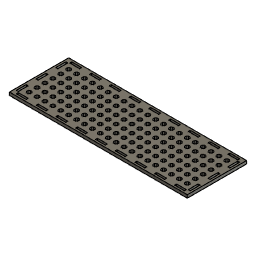
Modular Test Bench - Jumper Board v1 (Autodesk Fusion 360 design; units mm, degrees)
Autodesk Fusion 360 part; units mm, degrees
(part 1 of 2)
sketch "Sketch1" plane through (0, 0, 0) normal (0, 1, 0) x (1, 0, 0)
  line L0 (0, 0) -> (180, 0)
  line L1 (180, 0) -> (180, 60)
  line L2 (180, 60) -> (0, 60)
  line L3 (0, 60) -> (0, 0)
  dimension "d1" = 60
  dimension "d2" = 180
  constraint horizontal L0
  constraint vertical L1
  constraint horizontal L2
  constraint vertical L3
  constraint coincident L0.start L3.end
  measures "d1" distance of L0.start L2.end
  measures "d2" distance of L0.start L0.end
extrude "Extrude1" add sketch "Sketch1" along normal blind 3
sketch "Sketch2" plane through (0, 3, 0) normal (0, 1, 0) x (-1, 0, 0)
  line L0 (0, -60) -> (0, 0)
  line L1 (0, 0) -> (-180, 0)
  line L2 (-180, 0) -> (-180, -60)
  line L3 (-180, -60) -> (0, -60)
  line L4 (-5, -2) -> (-15, -2)
  line L5 (-15, -2) -> (-15, -4)
  line L6 (-15, -4) -> (-5, -4)
  line L7 (-5, -4) -> (-5, -2)
  line L8 (-25, -2) -> (-35, -2)
  line L9 (-25, -4) -> (-25, -2)
  line L10 (-35, -2) -> (-35, -4)
  line L11 (-35, -4) -> (-25, -4)
  line L12 (-45, -2) -> (-55, -2)
  line L13 (-45, -4) -> (-45, -2)
  line L14 (-55, -2) -> (-55, -4)
  line L15 (-55, -4) -> (-45, -4)
  line L16 (-65, -2) -> (-75, -2)
  line L17 (-65, -4) -> (-65, -2)
  line L18 (-75, -2) -> (-75, -4)
  line L19 (-75, -4) -> (-65, -4)
  line L20 (-85, -2) -> (-95, -2)
  line L21 (-85, -4) -> (-85, -2)
  line L22 (-95, -2) -> (-95, -4)
  line L23 (-95, -4) -> (-85, -4)
  line L24 (-105, -2) -> (-115, -2)
  line L25 (-105, -4) -> (-105, -2)
  line L26 (-115, -2) -> (-115, -4)
  line L27 (-115, -4) -> (-105, -4)
  line L28 (-125, -2) -> (-135, -2)
  line L29 (-125, -4) -> (-125, -2)
  line L30 (-135, -2) -> (-135, -4)
  line L31 (-135, -4) -> (-125, -4)
  line L32 (-145, -2) -> (-155, -2)
  line L33 (-145, -4) -> (-145, -2)
  line L34 (-155, -2) -> (-155, -4)
  line L35 (-155, -4) -> (-145, -4)
  line L36 (-165, -2) -> (-175, -2)
  line L37 (-165, -4) -> (-165, -2)
  line L38 (-175, -2) -> (-175, -4)
  line L39 (-175, -4) -> (-165, -4)
  line L40 (-5, -56) -> (-15, -56)
  line L41 (-5, -58) -> (-5, -56)
  line L42 (-15, -56) -> (-15, -58)
  line L43 (-15, -58) -> (-5, -58)
  line L44 (-25, -56) -> (-35, -56)
  line L45 (-25, -58) -> (-25, -56)
  line L46 (-35, -56) -> (-35, -58)
  line L47 (-35, -58) -> (-25, -58)
  line L48 (-45, -56) -> (-55, -56)
  line L49 (-45, -58) -> (-45, -56)
  line L50 (-55, -56) -> (-55, -58)
  line L51 (-55, -58) -> (-45, -58)
  line L52 (-65, -56) -> (-75, -56)
  line L53 (-65, -58) -> (-65, -56)
  line L54 (-75, -56) -> (-75, -58)
  line L55 (-75, -58) -> (-65, -58)
  line L56 (-85, -56) -> (-95, -56)
  line L57 (-85, -58) -> (-85, -56)
  line L58 (-95, -56) -> (-95, -58)
  line L59 (-95, -58) -> (-85, -58)
  line L60 (-105, -56) -> (-115, -56)
  line L61 (-105, -58) -> (-105, -56)
  line L62 (-115, -56) -> (-115, -58)
  line L63 (-115, -58) -> (-105, -58)
  line L64 (-125, -56) -> (-135, -56)
  line L65 (-125, -58) -> (-125, -56)
  line L66 (-135, -56) -> (-135, -58)
  line L67 (-135, -58) -> (-125, -58)
  line L68 (-145, -56) -> (-155, -56)
  line L69 (-145, -58) -> (-145, -56)
  line L70 (-155, -56) -> (-155, -58)
  line L71 (-155, -58) -> (-145, -58)
  line L72 (-165, -56) -> (-175, -56)
  line L73 (-165, -58) -> (-165, -56)
  line L74 (-175, -56) -> (-175, -58)
  line L75 (-175, -58) -> (-165, -58)
  line L76 (-2, -5) -> (-4, -5)
  line L77 (-4, -5) -> (-4, -15)
  line L78 (-4, -15) -> (-2, -15)
  line L79 (-2, -15) -> (-2, -5)
  line L80 (-178, -5) -> (-178, -15)
  line L81 (-176, -5) -> (-178, -5)
  line L82 (-176, -15) -> (-176, -5)
  line L83 (-178, -15) -> (-176, -15)
  line L84 (-4, -25) -> (-4, -35)
  line L85 (-2, -25) -> (-4, -25)
  line L86 (-2, -35) -> (-2, -25)
  line L87 (-4, -35) -> (-2, -35)
  line L88 (-178, -25) -> (-178, -35)
  line L89 (-176, -25) -> (-178, -25)
  line L90 (-176, -35) -> (-176, -25)
  line L91 (-178, -35) -> (-176, -35)
  line L92 (-4, -45) -> (-4, -55)
  line L93 (-2, -45) -> (-4, -45)
  line L94 (-2, -55) -> (-2, -45)
  line L95 (-4, -55) -> (-2, -55)
  line L96 (-178, -45) -> (-178, -55)
  line L97 (-176, -45) -> (-178, -45)
  line L98 (-176, -55) -> (-176, -45)
  line L99 (-178, -55) -> (-176, -55)
  line L100 (-12.0079, -50.8092) -> (-10.8476, -51.992)
  line L101 (-10.8476, -51.992) -> (-9.1908, -52.0079)
  line L102 (-9.1908, -52.0079) -> (-8.008, -50.8476)
  line L103 (-8.008, -50.8476) -> (-7.9921, -49.1908)
  line L104 (-7.9921, -49.1908) -> (-9.1524, -48.008)
  line L105 (-9.1524, -48.008) -> (-10.8092, -47.9921)
  line L106 (-10.8092, -47.9921) -> (-11.992, -49.1524)
  line L107 (-11.992, -49.1524) -> (-12.0079, -50.8092)
  line L108 (-18.8476, -51.992) -> (-17.1908, -52.0079)
  line L109 (-16.008, -50.8476) -> (-15.9921, -49.1908)
  line L110 (-15.9921, -49.1908) -> (-17.1524, -48.008)
  line L111 (-20.0079, -50.8092) -> (-18.8476, -51.992)
  line L112 (-17.1524, -48.008) -> (-18.8092, -47.9921)
  line L113 (-18.8092, -47.9921) -> (-19.992, -49.1524)
  line L114 (-19.992, -49.1524) -> (-20.0079, -50.8092)
  line L115 (-17.1908, -52.0079) -> (-16.008, -50.8476)
  line L116 (-26.8476, -51.992) -> (-25.1908, -52.0079)
  line L117 (-24.008, -50.8476) -> (-23.9921, -49.1908)
  line L118 (-23.9921, -49.1908) -> (-25.1524, -48.008)
  line L119 (-28.0079, -50.8092) -> (-26.8476, -51.992)
  line L120 (-25.1524, -48.008) -> (-26.8092, -47.9921)
  line L121 (-26.8092, -47.9921) -> (-27.992, -49.1524)
  line L122 (-27.992, -49.1524) -> (-28.0079, -50.8092)
  line L123 (-25.1908, -52.0079) -> (-24.008, -50.8476)
  line L124 (-34.8476, -51.992) -> (-33.1908, -52.0079)
  line L125 (-32.008, -50.8476) -> (-31.9921, -49.1908)
  line L126 (-31.9921, -49.1908) -> (-33.1524, -48.008)
  line L127 (-36.0079, -50.8092) -> (-34.8476, -51.992)
  line L128 (-33.1524, -48.008) -> (-34.8092, -47.9921)
  line L129 (-34.8092, -47.9921) -> (-35.992, -49.1524)
  line L130 (-35.992, -49.1524) -> (-36.0079, -50.8092)
  line L131 (-33.1908, -52.0079) -> (-32.008, -50.8476)
  line L132 (-42.8476, -51.992) -> (-41.1908, -52.0079)
  line L133 (-40.008, -50.8476) -> (-39.9921, -49.1908)
  line L134 (-39.9921, -49.1908) -> (-41.1524, -48.008)
  line L135 (-44.0079, -50.8092) -> (-42.8476, -51.992)
  line L136 (-41.1524, -48.008) -> (-42.8092, -47.9921)
  line L137 (-42.8092, -47.9921) -> (-43.992, -49.1524)
  line L138 (-43.992, -49.1524) -> (-44.0079, -50.8092)
  line L139 (-41.1908, -52.0079) -> (-40.008, -50.8476)
  line L140 (-50.8476, -51.992) -> (-49.1908, -52.0079)
  line L141 (-48.008, -50.8476) -> (-47.9921, -49.1908)
  line L142 (-47.9921, -49.1908) -> (-49.1524, -48.008)
  line L143 (-52.0079, -50.8092) -> (-50.8476, -51.992)
  line L144 (-49.1524, -48.008) -> (-50.8092, -47.9921)
  line L145 (-50.8092, -47.9921) -> (-51.992, -49.1524)
  line L146 (-51.992, -49.1524) -> (-52.0079, -50.8092)
  line L147 (-49.1908, -52.0079) -> (-48.008, -50.8476)
  line L148 (-58.8476, -51.992) -> (-57.1908, -52.0079)
  line L149 (-56.008, -50.8476) -> (-55.9921, -49.1908)
  line L150 (-55.9921, -49.1908) -> (-57.1524, -48.008)
  line L151 (-60.0079, -50.8092) -> (-58.8476, -51.992)
  line L152 (-57.1524, -48.008) -> (-58.8092, -47.9921)
  line L153 (-58.8092, -47.9921) -> (-59.992, -49.1524)
  line L154 (-59.992, -49.1524) -> (-60.0079, -50.8092)
  line L155 (-57.1908, -52.0079) -> (-56.008, -50.8476)
  line L156 (-66.8476, -51.992) -> (-65.1908, -52.0079)
  line L157 (-64.008, -50.8476) -> (-63.9921, -49.1908)
  line L158 (-63.9921, -49.1908) -> (-65.1524, -48.008)
  line L159 (-68.0079, -50.8092) -> (-66.8476, -51.992)
  line L160 (-65.1524, -48.008) -> (-66.8092, -47.9921)
  line L161 (-66.8092, -47.9921) -> (-67.992, -49.1524)
  line L162 (-67.992, -49.1524) -> (-68.0079, -50.8092)
  line L163 (-65.1908, -52.0079) -> (-64.008, -50.8476)
  line L164 (-74.8476, -51.992) -> (-73.1908, -52.0079)
  line L165 (-72.008, -50.8476) -> (-71.9921, -49.1908)
  line L166 (-71.9921, -49.1908) -> (-73.1524, -48.008)
  line L167 (-76.0079, -50.8092) -> (-74.8476, -51.992)
  line L168 (-73.1524, -48.008) -> (-74.8092, -47.9921)
  line L169 (-74.8092, -47.9921) -> (-75.992, -49.1524)
  line L170 (-75.992, -49.1524) -> (-76.0079, -50.8092)
  line L171 (-73.1908, -52.0079) -> (-72.008, -50.8476)
  line L172 (-82.8476, -51.992) -> (-81.1908, -52.0079)
  line L173 (-80.008, -50.8476) -> (-79.9921, -49.1908)
  line L174 (-79.9921, -49.1908) -> (-81.1524, -48.008)
  line L175 (-84.0079, -50.8092) -> (-82.8476, -51.992)
  line L176 (-81.1524, -48.008) -> (-82.8092, -47.9921)
  line L177 (-82.8092, -47.9921) -> (-83.992, -49.1524)
  line L178 (-83.992, -49.1524) -> (-84.0079, -50.8092)
  line L179 (-81.1908, -52.0079) -> (-80.008, -50.8476)
  line L180 (-90.8476, -51.992) -> (-89.1908, -52.0079)
  line L181 (-88.008, -50.8476) -> (-87.9921, -49.1908)
  line L182 (-87.9921, -49.1908) -> (-89.1524, -48.008)
  line L183 (-92.0079, -50.8092) -> (-90.8476, -51.992)
  line L184 (-89.1524, -48.008) -> (-90.8092, -47.9921)
  line L185 (-90.8092, -47.9921) -> (-91.992, -49.1524)
  line L186 (-91.992, -49.1524) -> (-92.0079, -50.8092)
  line L187 (-89.1908, -52.0079) -> (-88.008, -50.8476)
  line L188 (-98.8476, -51.992) -> (-97.1908, -52.0079)
  line L189 (-96.008, -50.8476) -> (-95.9921, -49.1908)
  line L190 (-95.9921, -49.1908) -> (-97.1524, -48.008)
  line L191 (-100.0079, -50.8092) -> (-98.8476, -51.992)
  line L192 (-97.1524, -48.008) -> (-98.8092, -47.9921)
  line L193 (-98.8092, -47.9921) -> (-99.992, -49.1524)
  line L194 (-99.992, -49.1524) -> (-100.0079, -50.8092)
  line L195 (-97.1908, -52.0079) -> (-96.008, -50.8476)
  line L196 (-106.8476, -51.992) -> (-105.1908, -52.0079)
  line L197 (-104.008, -50.8476) -> (-103.9921, -49.1908)
  line L198 (-103.9921, -49.1908) -> (-105.1524, -48.008)
  line L199 (-108.0079, -50.8092) -> (-106.8476, -51.992)
  line L200 (-105.1524, -48.008) -> (-106.8092, -47.9921)
  line L201 (-106.8092, -47.9921) -> (-107.992, -49.1524)
  line L202 (-107.992, -49.1524) -> (-108.0079, -50.8092)
  line L203 (-105.1908, -52.0079) -> (-104.008, -50.8476)
  line L204 (-114.8476, -51.992) -> (-113.1908, -52.0079)
  line L205 (-112.008, -50.8476) -> (-111.9921, -49.1908)
  line L206 (-111.9921, -49.1908) -> (-113.1524, -48.008)
  line L207 (-116.0079, -50.8092) -> (-114.8476, -51.992)
  line L208 (-113.1524, -48.008) -> (-114.8092, -47.9921)
  line L209 (-114.8092, -47.9921) -> (-115.992, -49.1524)
  line L210 (-115.992, -49.1524) -> (-116.0079, -50.8092)
  line L211 (-113.1908, -52.0079) -> (-112.008, -50.8476)
  line L212 (-122.8476, -51.992) -> (-121.1908, -52.0079)
  line L213 (-120.008, -50.8476) -> (-119.9921, -49.1908)
  line L214 (-119.9921, -49.1908) -> (-121.1524, -48.008)
  line L215 (-124.0079, -50.8092) -> (-122.8476, -51.992)
  line L216 (-121.1524, -48.008) -> (-122.8092, -47.9921)
  line L217 (-122.8092, -47.9921) -> (-123.992, -49.1524)
  line L218 (-123.992, -49.1524) -> (-124.0079, -50.8092)
  line L219 (-121.1908, -52.0079) -> (-120.008, -50.8476)
  line L220 (-130.8476, -51.992) -> (-129.1908, -52.0079)
  line L221 (-128.008, -50.8476) -> (-127.9921, -49.1908)
  line L222 (-127.9921, -49.1908) -> (-129.1524, -48.008)
  line L223 (-132.0079, -50.8092) -> (-130.8476, -51.992)
  line L224 (-129.1524, -48.008) -> (-130.8092, -47.9921)
  line L225 (-130.8092, -47.9921) -> (-131.992, -49.1524)
  line L226 (-131.992, -49.1524) -> (-132.0079, -50.8092)
  line L227 (-129.1908, -52.0079) -> (-128.008, -50.8476)
  line L228 (-138.8476, -51.992) -> (-137.1908, -52.0079)
  line L229 (-136.008, -50.8476) -> (-135.9921, -49.1908)
  line L230 (-135.9921, -49.1908) -> (-137.1524, -48.008)
  line L231 (-140.0079, -50.8092) -> (-138.8476, -51.992)
  line L232 (-137.1524, -48.008) -> (-138.8092, -47.9921)
  line L233 (-138.8092, -47.9921) -> (-139.992, -49.1524)
  line L234 (-139.992, -49.1524) -> (-140.0079, -50.8092)
  line L235 (-137.1908, -52.0079) -> (-136.008, -50.8476)
  line L236 (-146.8476, -51.992) -> (-145.1908, -52.0079)
  line L237 (-144.008, -50.8476) -> (-143.9921, -49.1908)
  line L238 (-143.9921, -49.1908) -> (-145.1524, -48.008)
  line L239 (-148.0079, -50.8092) -> (-146.8476, -51.992)
  line L240 (-145.1524, -48.008) -> (-146.8092, -47.9921)
  line L241 (-146.8092, -47.9921) -> (-147.992, -49.1524)
  line L242 (-147.992, -49.1524) -> (-148.0079, -50.8092)
  line L243 (-145.1908, -52.0079) -> (-144.008, -50.8476)
  line L244 (-154.8476, -51.992) -> (-153.1908, -52.0079)
  line L245 (-152.008, -50.8476) -> (-151.9921, -49.1908)
  line L246 (-151.9921, -49.1908) -> (-153.1524, -48.008)
  line L247 (-156.0079, -50.8092) -> (-154.8476, -51.992)
  line L248 (-153.1524, -48.008) -> (-154.8092, -47.9921)
  line L249 (-154.8092, -47.9921) -> (-155.992, -49.1524)
  line L250 (-155.992, -49.1524) -> (-156.0079, -50.8092)
  line L251 (-153.1908, -52.0079) -> (-152.008, -50.8476)
  line L252 (-162.8476, -51.992) -> (-161.1908, -52.0079)
  line L253 (-160.008, -50.8476) -> (-159.9921, -49.1908)
  line L254 (-159.9921, -49.1908) -> (-161.1524, -48.008)
  line L255 (-164.0079, -50.8092) -> (-162.8476, -51.992)
  line L256 (-161.1524, -48.008) -> (-162.8092, -47.9921)
  line L257 (-162.8092, -47.9921) -> (-163.992, -49.1524)
  line L258 (-163.992, -49.1524) -> (-164.0079, -50.8092)
  line L259 (-161.1908, -52.0079) -> (-160.008, -50.8476)
  line L260 (-170.8476, -51.992) -> (-169.1908, -52.0079)
  line L261 (-168.008, -50.8476) -> (-167.9921, -49.1908)
  line L262 (-167.9921, -49.1908) -> (-169.1524, -48.008)
  line L263 (-172.0079, -50.8092) -> (-170.8476, -51.992)
  line L264 (-169.1524, -48.008) -> (-170.8092, -47.9921)
  line L265 (-170.8092, -47.9921) -> (-171.992, -49.1524)
  line L266 (-171.992, -49.1524) -> (-172.0079, -50.8092)
  line L267 (-169.1908, -52.0079) -> (-168.008, -50.8476)
  line L268 (-10.8476, -43.992) -> (-9.1908, -44.0079)
  line L269 (-8.008, -42.8476) -> (-7.9921, -41.1908)
  line L270 (-7.9921, -41.1908) -> (-9.1524, -40.008)
  line L271 (-12.0079, -42.8092) -> (-10.8476, -43.992)
  line L272 (-9.1524, -40.008) -> (-10.8092, -39.9921)
  line L273 (-10.8092, -39.9921) -> (-11.992, -41.1524)
  line L274 (-11.992, -41.1524) -> (-12.0079, -42.8092)
  line L275 (-9.1908, -44.0079) -> (-8.008, -42.8476)
  line L276 (-18.8476, -43.992) -> (-17.1908, -44.0079)
  line L277 (-16.008, -42.8476) -> (-15.9921, -41.1908)
  line L278 (-15.9921, -41.1908) -> (-17.1524, -40.008)
  line L279 (-20.0079, -42.8092) -> (-18.8476, -43.992)
  line L280 (-17.1524, -40.008) -> (-18.8092, -39.9921)
  line L281 (-18.8092, -39.9921) -> (-19.992, -41.1524)
  line L282 (-19.992, -41.1524) -> (-20.0079, -42.8092)
  line L283 (-17.1908, -44.0079) -> (-16.008, -42.8476)
  line L284 (-26.8476, -43.992) -> (-25.1908, -44.0079)
  line L285 (-24.008, -42.8476) -> (-23.9921, -41.1908)
  line L286 (-23.9921, -41.1908) -> (-25.1524, -40.008)
  line L287 (-28.0079, -42.8092) -> (-26.8476, -43.992)
  line L288 (-25.1524, -40.008) -> (-26.8092, -39.9921)
  line L289 (-26.8092, -39.9921) -> (-27.992, -41.1524)
  line L290 (-27.992, -41.1524) -> (-28.0079, -42.8092)
  line L291 (-25.1908, -44.0079) -> (-24.008, -42.8476)
  line L292 (-34.8476, -43.992) -> (-33.1908, -44.0079)
  line L293 (-32.008, -42.8476) -> (-31.9921, -41.1908)
  line L294 (-31.9921, -41.1908) -> (-33.1524, -40.008)
  line L295 (-36.0079, -42.8092) -> (-34.8476, -43.992)
  line L296 (-33.1524, -40.008) -> (-34.8092, -39.9921)
  line L297 (-34.8092, -39.9921) -> (-35.992, -41.1524)
  line L298 (-35.992, -41.1524) -> (-36.0079, -42.8092)
  line L299 (-33.1908, -44.0079) -> (-32.008, -42.8476)
  line L300 (-42.8476, -43.992) -> (-41.1908, -44.0079)
  line L301 (-40.008, -42.8476) -> (-39.9921, -41.1908)
  line L302 (-39.9921, -41.1908) -> (-41.1524, -40.008)
  line L303 (-44.0079, -42.8092) -> (-42.8476, -43.992)
  line L304 (-41.1524, -40.008) -> (-42.8092, -39.9921)
  line L305 (-42.8092, -39.9921) -> (-43.992, -41.1524)
  line L306 (-43.992, -41.1524) -> (-44.0079, -42.8092)
  line L307 (-41.1908, -44.0079) -> (-40.008, -42.8476)
  line L308 (-50.8476, -43.992) -> (-49.1908, -44.0079)
  line L309 (-48.008, -42.8476) -> (-47.9921, -41.1908)
  line L310 (-47.9921, -41.1908) -> (-49.1524, -40.008)
  line L311 (-52.0079, -42.8092) -> (-50.8476, -43.992)
  line L312 (-49.1524, -40.008) -> (-50.8092, -39.9921)
  line L313 (-50.8092, -39.9921) -> (-51.992, -41.1524)
  line L314 (-51.992, -41.1524) -> (-52.0079, -42.8092)
  line L315 (-49.1908, -44.0079) -> (-48.008, -42.8476)
  line L316 (-58.8476, -43.992) -> (-57.1908, -44.0079)
  line L317 (-56.008, -42.8476) -> (-55.9921, -41.1908)
  line L318 (-55.9921, -41.1908) -> (-57.1524, -40.008)
  line L319 (-60.0079, -42.8092) -> (-58.8476, -43.992)
  line L320 (-57.1524, -40.008) -> (-58.8092, -39.9921)
  line L321 (-58.8092, -39.9921) -> (-59.992, -41.1524)
  line L322 (-59.992, -41.1524) -> (-60.0079, -42.8092)
  line L323 (-57.1908, -44.0079) -> (-56.008, -42.8476)
  line L324 (-66.8476, -43.992) -> (-65.1908, -44.0079)
  line L325 (-64.008, -42.8476) -> (-63.9921, -41.1908)
  line L326 (-63.9921, -41.1908) -> (-65.1524, -40.008)
  line L327 (-68.0079, -42.8092) -> (-66.8476, -43.992)
  line L328 (-65.1524, -40.008) -> (-66.8092, -39.9921)
  line L329 (-66.8092, -39.9921) -> (-67.992, -41.1524)
  line L330 (-67.992, -41.1524) -> (-68.0079, -42.8092)
  line L331 (-65.1908, -44.0079) -> (-64.008, -42.8476)
  line L332 (-74.8476, -43.992) -> (-73.1908, -44.0079)
  line L333 (-72.008, -42.8476) -> (-71.9921, -41.1908)
  line L334 (-71.9921, -41.1908) -> (-73.1524, -40.008)
  line L335 (-76.0079, -42.8092) -> (-74.8476, -43.992)
  line L336 (-73.1524, -40.008) -> (-74.8092, -39.9921)
  line L337 (-74.8092, -39.9921) -> (-75.992, -41.1524)
  line L338 (-75.992, -41.1524) -> (-76.0079, -42.8092)
  line L339 (-73.1908, -44.0079) -> (-72.008, -42.8476)
  line L340 (-82.8476, -43.992) -> (-81.1908, -44.0079)
  line L341 (-80.008, -42.8476) -> (-79.9921, -41.1908)
  line L342 (-79.9921, -41.1908) -> (-81.1524, -40.008)
  line L343 (-84.0079, -42.8092) -> (-82.8476, -43.992)
  line L344 (-81.1524, -40.008) -> (-82.8092, -39.9921)
  line L345 (-82.8092, -39.9921) -> (-83.992, -41.1524)
  line L346 (-83.992, -41.1524) -> (-84.0079, -42.8092)
  line L347 (-81.1908, -44.0079) -> (-80.008, -42.8476)
  line L348 (-90.8476, -43.992) -> (-89.1908, -44.0079)
  line L349 (-88.008, -42.8476) -> (-87.9921, -41.1908)
  line L350 (-87.9921, -41.1908) -> (-89.1524, -40.008)
  line L351 (-92.0079, -42.8092) -> (-90.8476, -43.992)
  line L352 (-89.1524, -40.008) -> (-90.8092, -39.9921)
  line L353 (-90.8092, -39.9921) -> (-91.992, -41.1524)
  line L354 (-91.992, -41.1524) -> (-92.0079, -42.8092)
  line L355 (-89.1908, -44.0079) -> (-88.008, -42.8476)
  line L356 (-98.8476, -43.992) -> (-97.1908, -44.0079)
  line L357 (-96.008, -42.8476) -> (-95.9921, -41.1908)
  line L358 (-95.9921, -41.1908) -> (-97.1524, -40.008)
  line L359 (-100.0079, -42.8092) -> (-98.8476, -43.992)
  line L360 (-97.1524, -40.008) -> (-98.8092, -39.9921)
  line L361 (-98.8092, -39.9921) -> (-99.992, -41.1524)
  line L362 (-99.992, -41.1524) -> (-100.0079, -42.8092)
  line L363 (-97.1908, -44.0079) -> (-96.008, -42.8476)
  line L364 (-106.8476, -43.992) -> (-105.1908, -44.0079)
  line L365 (-104.008, -42.8476) -> (-103.9921, -41.1908)
  line L366 (-103.9921, -41.1908) -> (-105.1524, -40.008)
  line L367 (-108.0079, -42.8092) -> (-106.8476, -43.992)
  line L368 (-105.1524, -40.008) -> (-106.8092, -39.9921)
  line L369 (-106.8092, -39.9921) -> (-107.992, -41.1524)
  line L370 (-107.992, -41.1524) -> (-108.0079, -42.8092)
  line L371 (-105.1908, -44.0079) -> (-104.008, -42.8476)
  line L372 (-114.8476, -43.992) -> (-113.1908, -44.0079)
  line L373 (-112.008, -42.8476) -> (-111.9921, -41.1908)
  line L374 (-111.9921, -41.1908) -> (-113.1524, -40.008)
  line L375 (-116.0079, -42.8092) -> (-114.8476, -43.992)
  line L376 (-113.1524, -40.008) -> (-114.8092, -39.9921)
  line L377 (-114.8092, -39.9921) -> (-115.992, -41.1524)
  line L378 (-115.992, -41.1524) -> (-116.0079, -42.8092)
  line L379 (-113.1908, -44.0079) -> (-112.008, -42.8476)
  line L380 (-122.8476, -43.992) -> (-121.1908, -44.0079)
  line L381 (-120.008, -42.8476) -> (-119.9921, -41.1908)
  line L382 (-119.9921, -41.1908) -> (-121.1524, -40.008)
  line L383 (-124.0079, -42.8092) -> (-122.8476, -43.992)
  line L384 (-121.1524, -40.008) -> (-122.8092, -39.9921)
  line L385 (-122.8092, -39.9921) -> (-123.992, -41.1524)
  line L386 (-123.992, -41.1524) -> (-124.0079, -42.8092)
  line L387 (-121.1908, -44.0079) -> (-120.008, -42.8476)
  line L388 (-130.8476, -43.992) -> (-129.1908, -44.0079)
  line L389 (-128.008, -42.8476) -> (-127.9921, -41.1908)
  line L390 (-127.9921, -41.1908) -> (-129.1524, -40.008)
  line L391 (-132.0079, -42.8092) -> (-130.8476, -43.992)
  line L392 (-129.1524, -40.008) -> (-130.8092, -39.9921)
  line L393 (-130.8092, -39.9921) -> (-131.992, -41.1524)
  line L394 (-131.992, -41.1524) -> (-132.0079, -42.8092)
  line L395 (-129.1908, -44.0079) -> (-128.008, -42.8476)
  line L396 (-138.8476, -43.992) -> (-137.1908, -44.0079)
  line L397 (-136.008, -42.8476) -> (-135.9921, -41.1908)
  line L398 (-135.9921, -41.1908) -> (-137.1524, -40.008)
  line L399 (-140.0079, -42.8092) -> (-138.8476, -43.992)
  line L400 (-137.1524, -40.008) -> (-138.8092, -39.9921)
  line L401 (-138.8092, -39.9921) -> (-139.992, -41.1524)
  line L402 (-139.992, -41.1524) -> (-140.0079, -42.8092)
  line L403 (-137.1908, -44.0079) -> (-136.008, -42.8476)
  line L404 (-146.8476, -43.992) -> (-145.1908, -44.0079)
  line L405 (-144.008, -42.8476) -> (-143.9921, -41.1908)
  line L406 (-143.9921, -41.1908) -> (-145.1524, -40.008)
  line L407 (-148.0079, -42.8092) -> (-146.8476, -43.992)
  line L408 (-145.1524, -40.008) -> (-146.8092, -39.9921)
  line L409 (-146.8092, -39.9921) -> (-147.992, -41.1524)
  line L410 (-147.992, -41.1524) -> (-148.0079, -42.8092)
  line L411 (-145.1908, -44.0079) -> (-144.008, -42.8476)
  line L412 (-154.8476, -43.992) -> (-153.1908, -44.0079)
  line L413 (-152.008, -42.8476) -> (-151.9921, -41.1908)
  line L414 (-151.9921, -41.1908) -> (-153.1524, -40.008)
  line L415 (-156.0079, -42.8092) -> (-154.8476, -43.992)
  line L416 (-153.1524, -40.008) -> (-154.8092, -39.9921)
  line L417 (-154.8092, -39.9921) -> (-155.992, -41.1524)
  line L418 (-155.992, -41.1524) -> (-156.0079, -42.8092)
  line L419 (-153.1908, -44.0079) -> (-152.008, -42.8476)
  line L420 (-162.8476, -43.992) -> (-161.1908, -44.0079)
  line L421 (-160.008, -42.8476) -> (-159.9921, -41.1908)
  line L422 (-159.9921, -41.1908) -> (-161.1524, -40.008)
  line L423 (-164.0079, -42.8092) -> (-162.8476, -43.992)
  line L424 (-161.1524, -40.008) -> (-162.8092, -39.9921)
  line L425 (-162.8092, -39.9921) -> (-163.992, -41.1524)
  line L426 (-163.992, -41.1524) -> (-164.0079, -42.8092)
  line L427 (-161.1908, -44.0079) -> (-160.008, -42.8476)
  line L428 (-170.8476, -43.992) -> (-169.1908, -44.0079)
  line L429 (-168.008, -42.8476) -> (-167.9921, -41.1908)
  line L430 (-167.9921, -41.1908) -> (-169.1524, -40.008)
  line L431 (-172.0079, -42.8092) -> (-170.8476, -43.992)
  line L432 (-169.1524, -40.008) -> (-170.8092, -39.9921)
  line L433 (-170.8092, -39.9921) -> (-171.992, -41.1524)
  line L434 (-171.992, -41.1524) -> (-172.0079, -42.8092)
  line L435 (-169.1908, -44.0079) -> (-168.008, -42.8476)
  line L436 (-10.8476, -35.992) -> (-9.1908, -36.0079)
  line L437 (-8.008, -34.8476) -> (-7.9921, -33.1908)
  line L438 (-7.9921, -33.1908) -> (-9.1524, -32.008)
  line L439 (-12.0079, -34.8092) -> (-10.8476, -35.992)
  line L440 (-9.1524, -32.008) -> (-10.8092, -31.9921)
  line L441 (-10.8092, -31.9921) -> (-11.992, -33.1524)
  line L442 (-11.992, -33.1524) -> (-12.0079, -34.8092)
  line L443 (-9.1908, -36.0079) -> (-8.008, -34.8476)
  line L444 (-18.8476, -35.992) -> (-17.1908, -36.0079)
  line L445 (-16.008, -34.8476) -> (-15.9921, -33.1908)
  line L446 (-15.9921, -33.1908) -> (-17.1524, -32.008)
  line L447 (-20.0079, -34.8092) -> (-18.8476, -35.992)
  line L448 (-17.1524, -32.008) -> (-18.8092, -31.9921)
  line L449 (-18.8092, -31.9921) -> (-19.992, -33.1524)
  line L450 (-19.992, -33.1524) -> (-20.0079, -34.8092)
  line L451 (-17.1908, -36.0079) -> (-16.008, -34.8476)
  line L452 (-26.8476, -35.992) -> (-25.1908, -36.0079)
  line L453 (-24.008, -34.8476) -> (-23.9921, -33.1908)
  line L454 (-23.9921, -33.1908) -> (-25.1524, -32.008)
  line L455 (-28.0079, -34.8092) -> (-26.8476, -35.992)
  line L456 (-25.1524, -32.008) -> (-26.8092, -31.9921)
  line L457 (-26.8092, -31.9921) -> (-27.992, -33.1524)
  line L458 (-27.992, -33.1524) -> (-28.0079, -34.8092)
  line L459 (-25.1908, -36.0079) -> (-24.008, -34.8476)
  line L460 (-34.8476, -35.992) -> (-33.1908, -36.0079)
  line L461 (-32.008, -34.8476) -> (-31.9921, -33.1908)
  line L462 (-31.9921, -33.1908) -> (-33.1524, -32.008)
  line L463 (-36.0079, -34.8092) -> (-34.8476, -35.992)
  line L464 (-33.1524, -32.008) -> (-34.8092, -31.9921)
  line L465 (-34.8092, -31.9921) -> (-35.992, -33.1524)
  line L466 (-35.992, -33.1524) -> (-36.0079, -34.8092)
  line L467 (-33.1908, -36.0079) -> (-32.008, -34.8476)
  line L468 (-42.8476, -35.992) -> (-41.1908, -36.0079)
  line L469 (-40.008, -34.8476) -> (-39.9921, -33.1908)
  line L470 (-39.9921, -33.1908) -> (-41.1524, -32.008)
  line L471 (-44.0079, -34.8092) -> (-42.8476, -35.992)
  line L472 (-41.1524, -32.008) -> (-42.8092, -31.9921)
  line L473 (-42.8092, -31.9921) -> (-43.992, -33.1524)
  line L474 (-43.992, -33.1524) -> (-44.0079, -34.8092)
  line L475 (-41.1908, -36.0079) -> (-40.008, -34.8476)
  line L476 (-50.8476, -35.992) -> (-49.1908, -36.0079)
  line L477 (-48.008, -34.8476) -> (-47.9921, -33.1908)
  line L478 (-47.9921, -33.1908) -> (-49.1524, -32.008)
  line L479 (-52.0079, -34.8092) -> (-50.8476, -35.992)
  line L480 (-49.1524, -32.008) -> (-50.8092, -31.9921)
  line L481 (-50.8092, -31.9921) -> (-51.992, -33.1524)
  line L482 (-51.992, -33.1524) -> (-52.0079, -34.8092)
  line L483 (-49.1908, -36.0079) -> (-48.008, -34.8476)
  line L484 (-58.8476, -35.992) -> (-57.1908, -36.0079)
  line L485 (-56.008, -34.8476) -> (-55.9921, -33.1908)
  line L486 (-55.9921, -33.1908) -> (-57.1524, -32.008)
  line L487 (-60.0079, -34.8092) -> (-58.8476, -35.992)
  line L488 (-57.1524, -32.008) -> (-58.8092, -31.9921)
  line L489 (-58.8092, -31.9921) -> (-59.992, -33.1524)
  line L490 (-59.992, -33.1524) -> (-60.0079, -34.8092)
  line L491 (-57.1908, -36.0079) -> (-56.008, -34.8476)
  line L492 (-66.8476, -35.992) -> (-65.1908, -36.0079)
  line L493 (-64.008, -34.8476) -> (-63.9921, -33.1908)
  line L494 (-63.9921, -33.1908) -> (-65.1524, -32.008)
  line L495 (-68.0079, -34.8092) -> (-66.8476, -35.992)
  line L496 (-65.1524, -32.008) -> (-66.8092, -31.9921)
  line L497 (-66.8092, -31.9921) -> (-67.992, -33.1524)
  line L498 (-67.992, -33.1524) -> (-68.0079, -34.8092)
  line L499 (-65.1908, -36.0079) -> (-64.008, -34.8476)
  line L500 (-74.8476, -35.992) -> (-73.1908, -36.0079)
  line L501 (-72.008, -34.8476) -> (-71.9921, -33.1908)
  line L502 (-71.9921, -33.1908) -> (-73.1524, -32.008)
  line L503 (-76.0079, -34.8092) -> (-74.8476, -35.992)
  line L504 (-73.1524, -32.008) -> (-74.8092, -31.9921)
  line L505 (-74.8092, -31.9921) -> (-75.992, -33.1524)
  line L506 (-75.992, -33.1524) -> (-76.0079, -34.8092)
  line L507 (-73.1908, -36.0079) -> (-72.008, -34.8476)
  line L508 (-82.8476, -35.992) -> (-81.1908, -36.0079)
  line L509 (-80.008, -34.8476) -> (-79.9921, -33.1908)
  line L510 (-79.9921, -33.1908) -> (-81.1524, -32.008)
  line L511 (-84.0079, -34.8092) -> (-82.8476, -35.992)
  line L512 (-81.1524, -32.008) -> (-82.8092, -31.9921)
  line L513 (-82.8092, -31.9921) -> (-83.992, -33.1524)
  line L514 (-83.992, -33.1524) -> (-84.0079, -34.8092)
  line L515 (-81.1908, -36.0079) -> (-80.008, -34.8476)
  line L516 (-90.8476, -35.992) -> (-89.1908, -36.0079)
  line L517 (-88.008, -34.8476) -> (-87.9921, -33.1908)
  line L518 (-87.9921, -33.1908) -> (-89.1524, -32.008)
  line L519 (-92.0079, -34.8092) -> (-90.8476, -35.992)
  line L520 (-89.1524, -32.008) -> (-90.8092, -31.9921)
  line L521 (-90.8092, -31.9921) -> (-91.992, -33.1524)
  line L522 (-91.992, -33.1524) -> (-92.0079, -34.8092)
  line L523 (-89.1908, -36.0079) -> (-88.008, -34.8476)
  line L524 (-98.8476, -35.992) -> (-97.1908, -36.0079)
  line L525 (-96.008, -34.8476) -> (-95.9921, -33.1908)
  line L526 (-95.9921, -33.1908) -> (-97.1524, -32.008)
  line L527 (-100.0079, -34.8092) -> (-98.8476, -35.992)
  line L528 (-97.1524, -32.008) -> (-98.8092, -31.9921)
  line L529 (-98.8092, -31.9921) -> (-99.992, -33.1524)
  line L530 (-99.992, -33.1524) -> (-100.0079, -34.8092)
  line L531 (-97.1908, -36.0079) -> (-96.008, -34.8476)
  line L532 (-106.8476, -35.992) -> (-105.1908, -36.0079)
  line L533 (-104.008, -34.8476) -> (-103.9921, -33.1908)
  line L534 (-103.9921, -33.1908) -> (-105.1524, -32.008)
  line L535 (-108.0079, -34.8092) -> (-106.8476, -35.992)
  line L536 (-105.1524, -32.008) -> (-106.8092, -31.9921)
  line L537 (-106.8092, -31.9921) -> (-107.992, -33.1524)
  line L538 (-107.992, -33.1524) -> (-108.0079, -34.8092)
  line L539 (-105.1908, -36.0079) -> (-104.008, -34.8476)
  line L540 (-114.8476, -35.992) -> (-113.1908, -36.0079)
  line L541 (-112.008, -34.8476) -> (-111.9921, -33.1908)
  line L542 (-111.9921, -33.1908) -> (-113.1524, -32.008)
  line L543 (-116.0079, -34.8092) -> (-114.8476, -35.992)
  line L544 (-113.1524, -32.008) -> (-114.8092, -31.9921)
  line L545 (-114.8092, -31.9921) -> (-115.992, -33.1524)
  line L546 (-115.992, -33.1524) -> (-116.0079, -34.8092)
  line L547 (-113.1908, -36.0079) -> (-112.008, -34.8476)
  line L548 (-122.8476, -35.992) -> (-121.1908, -36.0079)
  line L549 (-120.008, -34.8476) -> (-119.9921, -33.1908)
  line L550 (-119.9921, -33.1908) -> (-121.1524, -32.008)
  line L551 (-124.0079, -34.8092) -> (-122.8476, -35.992)
  line L552 (-121.1524, -32.008) -> (-122.8092, -31.9921)
  line L553 (-122.8092, -31.9921) -> (-123.992, -33.1524)
  line L554 (-123.992, -33.1524) -> (-124.0079, -34.8092)
  line L555 (-121.1908, -36.0079) -> (-120.008, -34.8476)
  line L556 (-130.8476, -35.992) -> (-129.1908, -36.0079)
  line L557 (-128.008, -34.8476) -> (-127.9921, -33.1908)
  line L558 (-127.9921, -33.1908) -> (-129.1524, -32.008)
  line L559 (-132.0079, -34.8092) -> (-130.8476, -35.992)
  line L560 (-129.1524, -32.008) -> (-130.8092, -31.9921)
  line L561 (-130.8092, -31.9921) -> (-131.992, -33.1524)
  line L562 (-131.992, -33.1524) -> (-132.0079, -34.8092)
  line L563 (-129.1908, -36.0079) -> (-128.008, -34.8476)
  line L564 (-138.8476, -35.992) -> (-137.1908, -36.0079)
  line L565 (-136.008, -34.8476) -> (-135.9921, -33.1908)
  line L566 (-135.9921, -33.1908) -> (-137.1524, -32.008)
  line L567 (-140.0079, -34.8092) -> (-138.8476, -35.992)
  line L568 (-137.1524, -32.008) -> (-138.8092, -31.9921)
  line L569 (-138.8092, -31.9921) -> (-139.992, -33.1524)
  line L570 (-139.992, -33.1524) -> (-140.0079, -34.8092)
  line L571 (-137.1908, -36.0079) -> (-136.008, -34.8476)
  line L572 (-146.8476, -35.992) -> (-145.1908, -36.0079)
  line L573 (-144.008, -34.8476) -> (-143.9921, -33.1908)
  line L574 (-143.9921, -33.1908) -> (-145.1524, -32.008)
  line L575 (-148.0079, -34.8092) -> (-146.8476, -35.992)
  line L576 (-145.1524, -32.008) -> (-146.8092, -31.9921)
  line L577 (-146.8092, -31.9921) -> (-147.992, -33.1524)
  line L578 (-147.992, -33.1524) -> (-148.0079, -34.8092)
  line L579 (-145.1908, -36.0079) -> (-144.008, -34.8476)
  line L580 (-154.8476, -35.992) -> (-153.1908, -36.0079)
  line L581 (-152.008, -34.8476) -> (-151.9921, -33.1908)
  line L582 (-151.9921, -33.1908) -> (-153.1524, -32.008)
  line L583 (-156.0079, -34.8092) -> (-154.8476, -35.992)
  line L584 (-153.1524, -32.008) -> (-154.8092, -31.9921)
  line L585 (-154.8092, -31.9921) -> (-155.992, -33.1524)
  line L586 (-155.992, -33.1524) -> (-156.0079, -34.8092)
  line L587 (-153.1908, -36.0079) -> (-152.008, -34.8476)
  line L588 (-162.8476, -35.992) -> (-161.1908, -36.0079)
  line L589 (-160.008, -34.8476) -> (-159.9921, -33.1908)
  line L590 (-159.9921, -33.1908) -> (-161.1524, -32.008)
  line L591 (-164.0079, -34.8092) -> (-162.8476, -35.992)
  line L592 (-161.1524, -32.008) -> (-162.8092, -31.9921)
  line L593 (-162.8092, -31.9921) -> (-163.992, -33.1524)
  line L594 (-163.992, -33.1524) -> (-164.0079, -34.8092)
  line L595 (-161.1908, -36.0079) -> (-160.008, -34.8476)
  line L596 (-170.8476, -35.992) -> (-169.1908, -36.0079)
  line L597 (-168.008, -34.8476) -> (-167.9921, -33.1908)
  line L598 (-167.9921, -33.1908) -> (-169.1524, -32.008)
  line L599 (-172.0079, -34.8092) -> (-170.8476, -35.992)
  line L600 (-169.1524, -32.008) -> (-170.8092, -31.9921)
  line L601 (-170.8092, -31.9921) -> (-171.992, -33.1524)
  line L602 (-171.992, -33.1524) -> (-172.0079, -34.8092)
  line L603 (-169.1908, -36.0079) -> (-168.008, -34.8476)
  line L604 (-10.8476, -27.992) -> (-9.1908, -28.0079)
  line L605 (-8.008, -26.8476) -> (-7.9921, -25.1908)
  line L606 (-7.9921, -25.1908) -> (-9.1524, -24.008)
  line L607 (-12.0079, -26.8092) -> (-10.8476, -27.992)
  line L608 (-9.1524, -24.008) -> (-10.8092, -23.9921)
  line L609 (-10.8092, -23.9921) -> (-11.992, -25.1524)
  line L610 (-11.992, -25.1524) -> (-12.0079, -26.8092)
  line L611 (-9.1908, -28.0079) -> (-8.008, -26.8476)
  line L612 (-18.8476, -27.992) -> (-17.1908, -28.0079)
  line L613 (-16.008, -26.8476) -> (-15.9921, -25.1908)
  line L614 (-15.9921, -25.1908) -> (-17.1524, -24.008)
  line L615 (-20.0079, -26.8092) -> (-18.8476, -27.992)
  line L616 (-17.1524, -24.008) -> (-18.8092, -23.9921)
  line L617 (-18.8092, -23.9921) -> (-19.992, -25.1524)
  line L618 (-19.992, -25.1524) -> (-20.0079, -26.8092)
  line L619 (-17.1908, -28.0079) -> (-16.008, -26.8476)
  line L620 (-26.8476, -27.992) -> (-25.1908, -28.0079)
  line L621 (-24.008, -26.8476) -> (-23.9921, -25.1908)
  line L622 (-23.9921, -25.1908) -> (-25.1524, -24.008)
  line L623 (-28.0079, -26.8092) -> (-26.8476, -27.992)
  line L624 (-25.1524, -24.008) -> (-26.8092, -23.9921)
  line L625 (-26.8092, -23.9921) -> (-27.992, -25.1524)
  line L626 (-27.992, -25.1524) -> (-28.0079, -26.8092)
  line L627 (-25.1908, -28.0079) -> (-24.008, -26.8476)
  line L628 (-34.8476, -27.992) -> (-33.1908, -28.0079)
  line L629 (-32.008, -26.8476) -> (-31.9921, -25.1908)
  line L630 (-31.9921, -25.1908) -> (-33.1524, -24.008)
  line L631 (-36.0079, -26.8092) -> (-34.8476, -27.992)
  line L632 (-33.1524, -24.008) -> (-34.8092, -23.9921)
  line L633 (-34.8092, -23.9921) -> (-35.992, -25.1524)
  line L634 (-35.992, -25.1524) -> (-36.0079, -26.8092)
  line L635 (-33.1908, -28.0079) -> (-32.008, -26.8476)
  line L636 (-42.8476, -27.992) -> (-41.1908, -28.0079)
  line L637 (-40.008, -26.8476) -> (-39.9921, -25.1908)
  line L638 (-39.9921, -25.1908) -> (-41.1524, -24.008)
  line L639 (-44.0079, -26.8092) -> (-42.8476, -27.992)
  line L640 (-41.1524, -24.008) -> (-42.8092, -23.9921)
  line L641 (-42.8092, -23.9921) -> (-43.992, -25.1524)
  line L642 (-43.992, -25.1524) -> (-44.0079, -26.8092)
  line L643 (-41.1908, -28.0079) -> (-40.008, -26.8476)
  line L644 (-50.8476, -27.992) -> (-49.1908, -28.0079)
  line L645 (-48.008, -26.8476) -> (-47.9921, -25.1908)
  line L646 (-47.9921, -25.1908) -> (-49.1524, -24.008)
  line L647 (-52.0079, -26.8092) -> (-50.8476, -27.992)
  line L648 (-49.1524, -24.008) -> (-50.8092, -23.9921)
  line L649 (-50.8092, -23.9921) -> (-51.992, -25.1524)
  line L650 (-51.992, -25.1524) -> (-52.0079, -26.8092)
  line L651 (-49.1908, -28.0079) -> (-48.008, -26.8476)
  line L652 (-58.8476, -27.992) -> (-57.1908, -28.0079)
  line L653 (-56.008, -26.8476) -> (-55.9921, -25.1908)
  line L654 (-55.9921, -25.1908) -> (-57.1524, -24.008)
  line L655 (-60.0079, -26.8092) -> (-58.8476, -27.992)
  line L656 (-57.1524, -24.008) -> (-58.8092, -23.9921)
  line L657 (-58.8092, -23.9921) -> (-59.992, -25.1524)
  line L658 (-59.992, -25.1524) -> (-60.0079, -26.8092)
  line L659 (-57.1908, -28.0079) -> (-56.008, -26.8476)
  line L660 (-66.8476, -27.992) -> (-65.1908, -28.0079)
  line L661 (-64.008, -26.8476) -> (-63.9921, -25.1908)
  line L662 (-63.9921, -25.1908) -> (-65.1524, -24.008)
  line L663 (-68.0079, -26.8092) -> (-66.8476, -27.992)
  line L664 (-65.1524, -24.008) -> (-66.8092, -23.9921)
  line L665 (-66.8092, -23.9921) -> (-67.992, -25.1524)
  line L666 (-67.992, -25.1524) -> (-68.0079, -26.8092)
  line L667 (-65.1908, -28.0079) -> (-64.008, -26.8476)
  line L668 (-74.8476, -27.992) -> (-73.1908, -28.0079)
  line L669 (-72.008, -26.8476) -> (-71.9921, -25.1908)
  line L670 (-71.9921, -25.1908) -> (-73.1524, -24.008)
  line L671 (-76.0079, -26.8092) -> (-74.8476, -27.992)
  line L672 (-73.1524, -24.008) -> (-74.8092, -23.9921)
  line L673 (-74.8092, -23.9921) -> (-75.992, -25.1524)
  line L674 (-75.992, -25.1524) -> (-76.0079, -26.8092)
  line L675 (-73.1908, -28.0079) -> (-72.008, -26.8476)
  line L676 (-82.8476, -27.992) -> (-81.1908, -28.0079)
  line L677 (-80.008, -26.8476) -> (-79.9921, -25.1908)
  line L678 (-79.9921, -25.1908) -> (-81.1524, -24.008)
  line L679 (-84.0079, -26.8092) -> (-82.8476, -27.992)
  line L680 (-81.1524, -24.008) -> (-82.8092, -23.9921)
  line L681 (-82.8092, -23.9921) -> (-83.992, -25.1524)
  line L682 (-83.992, -25.1524) -> (-84.0079, -26.8092)
  line L683 (-81.1908, -28.0079) -> (-80.008, -26.8476)
  line L684 (-90.8476, -27.992) -> (-89.1908, -28.0079)
  line L685 (-88.008, -26.8476) -> (-87.9921, -25.1908)
  line L686 (-87.9921, -25.1908) -> (-89.1524, -24.008)
  line L687 (-92.0079, -26.8092) -> (-90.8476, -27.992)
  line L688 (-89.1524, -24.008) -> (-90.8092, -23.9921)
  line L689 (-90.8092, -23.9921) -> (-91.992, -25.1524)
  line L690 (-91.992, -25.1524) -> (-92.0079, -26.8092)
  line L691 (-89.1908, -28.0079) -> (-88.008, -26.8476)
  line L692 (-98.8476, -27.992) -> (-97.1908, -28.0079)
  line L693 (-96.008, -26.8476) -> (-95.9921, -25.1908)
  line L694 (-95.9921, -25.1908) -> (-97.1524, -24.008)
  line L695 (-100.0079, -26.8092) -> (-98.8476, -27.992)
  line L696 (-97.1524, -24.008) -> (-98.8092, -23.9921)
  line L697 (-98.8092, -23.9921) -> (-99.992, -25.1524)
  line L698 (-99.992, -25.1524) -> (-100.0079, -26.8092)
  line L699 (-97.1908, -28.0079) -> (-96.008, -26.8476)
  line L700 (-106.8476, -27.992) -> (-105.1908, -28.0079)
  line L701 (-104.008, -26.8476) -> (-103.9921, -25.1908)
  line L702 (-103.9921, -25.1908) -> (-105.1524, -24.008)
  line L703 (-108.0079, -26.8092) -> (-106.8476, -27.992)
  line L704 (-105.1524, -24.008) -> (-106.8092, -23.9921)
  line L705 (-106.8092, -23.9921) -> (-107.992, -25.1524)
  line L706 (-107.992, -25.1524) -> (-108.0079, -26.8092)
  line L707 (-105.1908, -28.0079) -> (-104.008, -26.8476)
  line L708 (-114.8476, -27.992) -> (-113.1908, -28.0079)
  line L709 (-112.008, -26.8476) -> (-111.9921, -25.1908)
  line L710 (-111.9921, -25.1908) -> (-113.1524, -24.008)
  line L711 (-116.0079, -26.8092) -> (-114.8476, -27.992)
  line L712 (-113.1524, -24.008) -> (-114.8092, -23.9921)
  line L713 (-114.8092, -23.9921) -> (-115.992, -25.1524)
  line L714 (-115.992, -25.1524) -> (-116.0079, -26.8092)
  line L715 (-113.1908, -28.0079) -> (-112.008, -26.8476)
  line L716 (-122.8476, -27.992) -> (-121.1908, -28.0079)
  line L717 (-120.008, -26.8476) -> (-119.9921, -25.1908)
  line L718 (-119.9921, -25.1908) -> (-121.1524, -24.008)
  line L719 (-124.0079, -26.8092) -> (-122.8476, -27.992)
  line L720 (-121.1524, -24.008) -> (-122.8092, -23.9921)
  line L721 (-122.8092, -23.9921) -> (-123.992, -25.1524)
  line L722 (-123.992, -25.1524) -> (-124.0079, -26.8092)
  line L723 (-121.1908, -28.0079) -> (-120.008, -26.8476)
  line L724 (-130.8476, -27.992) -> (-129.1908, -28.0079)
  line L725 (-128.008, -26.8476) -> (-127.9921, -25.1908)
  line L726 (-127.9921, -25.1908) -> (-129.1524, -24.008)
  line L727 (-132.0079, -26.8092) -> (-130.8476, -27.992)
  line L728 (-129.1524, -24.008) -> (-130.8092, -23.9921)
  line L729 (-130.8092, -23.9921) -> (-131.992, -25.1524)
  line L730 (-131.992, -25.1524) -> (-132.0079, -26.8092)
  line L731 (-129.1908, -28.0079) -> (-128.008, -26.8476)
  line L732 (-138.8476, -27.992) -> (-137.1908, -28.0079)
  line L733 (-136.008, -26.8476) -> (-135.9921, -25.1908)
  line L734 (-135.9921, -25.1908) -> (-137.1524, -24.008)
  line L735 (-140.0079, -26.8092) -> (-138.8476, -27.992)
  line L736 (-137.1524, -24.008) -> (-138.8092, -23.9921)
  line L737 (-138.8092, -23.9921) -> (-139.992, -25.1524)
  line L738 (-139.992, -25.1524) -> (-140.0079, -26.8092)
  line L739 (-137.1908, -28.0079) -> (-136.008, -26.8476)
  line L740 (-146.8476, -27.992) -> (-145.1908, -28.0079)
  line L741 (-144.008, -26.8476) -> (-143.9921, -25.1908)
  line L742 (-143.9921, -25.1908) -> (-145.1524, -24.008)
  line L743 (-148.0079, -26.8092) -> (-146.8476, -27.992)
  line L744 (-145.1524, -24.008) -> (-146.8092, -23.9921)
  line L745 (-146.8092, -23.9921) -> (-147.992, -25.1524)
  line L746 (-147.992, -25.1524) -> (-148.0079, -26.8092)
  line L747 (-145.1908, -28.0079) -> (-144.008, -26.8476)
  line L748 (-154.8476, -27.992) -> (-153.1908, -28.0079)
  line L749 (-152.008, -26.8476) -> (-151.9921, -25.1908)
  line L750 (-151.9921, -25.1908) -> (-153.1524, -24.008)
  line L751 (-156.0079, -26.8092) -> (-154.8476, -27.992)
  line L752 (-153.1524, -24.008) -> (-154.8092, -23.9921)
  line L753 (-154.8092, -23.9921) -> (-155.992, -25.1524)
  line L754 (-155.992, -25.1524) -> (-156.0079, -26.8092)
  line L755 (-153.1908, -28.0079) -> (-152.008, -26.8476)
  line L756 (-162.8476, -27.992) -> (-161.1908, -28.0079)
  line L757 (-160.008, -26.8476) -> (-159.9921, -25.1908)
  line L758 (-159.9921, -25.1908) -> (-161.1524, -24.008)
  line L759 (-164.0079, -26.8092) -> (-162.8476, -27.992)
  line L760 (-161.1524, -24.008) -> (-162.8092, -23.9921)
  line L761 (-162.8092, -23.9921) -> (-163.992, -25.1524)
  line L762 (-163.992, -25.1524) -> (-164.0079, -26.8092)
  line L763 (-161.1908, -28.0079) -> (-160.008, -26.8476)
  line L764 (-170.8476, -27.992) -> (-169.1908, -28.0079)
  line L765 (-168.008, -26.8476) -> (-167.9921, -25.1908)
  line L766 (-167.9921, -25.1908) -> (-169.1524, -24.008)
  line L767 (-172.0079, -26.8092) -> (-170.8476, -27.992)
  line L768 (-169.1524, -24.008) -> (-170.8092, -23.9921)
  line L769 (-170.8092, -23.9921) -> (-171.992, -25.1524)
  line L770 (-171.992, -25.1524) -> (-172.0079, -26.8092)
  line L771 (-169.1908, -28.0079) -> (-168.008, -26.8476)
  line L772 (-10.8476, -19.992) -> (-9.1908, -20.0079)
  line L773 (-8.008, -18.8476) -> (-7.9921, -17.1908)
  line L774 (-7.9921, -17.1908) -> (-9.1524, -16.008)
  line L775 (-12.0079, -18.8092) -> (-10.8476, -19.992)
  line L776 (-9.1524, -16.008) -> (-10.8092, -15.9921)
  line L777 (-10.8092, -15.9921) -> (-11.992, -17.1524)
  line L778 (-11.992, -17.1524) -> (-12.0079, -18.8092)
  line L779 (-9.1908, -20.0079) -> (-8.008, -18.8476)
  line L780 (-18.8476, -19.992) -> (-17.1908, -20.0079)
  line L781 (-16.008, -18.8476) -> (-15.9921, -17.1908)
  line L782 (-15.9921, -17.1908) -> (-17.1524, -16.008)
  line L783 (-20.0079, -18.8092) -> (-18.8476, -19.992)
  line L784 (-17.1524, -16.008) -> (-18.8092, -15.9921)
  line L785 (-18.8092, -15.9921) -> (-19.992, -17.1524)
  line L786 (-19.992, -17.1524) -> (-20.0079, -18.8092)
  line L787 (-17.1908, -20.0079) -> (-16.008, -18.8476)
  line L788 (-26.8476, -19.992) -> (-25.1908, -20.0079)
  line L789 (-24.008, -18.8476) -> (-23.9921, -17.1908)
  line L790 (-23.9921, -17.1908) -> (-25.1524, -16.008)
  line L791 (-28.0079, -18.8092) -> (-26.8476, -19.992)
  line L792 (-25.1524, -16.008) -> (-26.8092, -15.9921)
  line L793 (-26.8092, -15.9921) -> (-27.992, -17.1524)
  line L794 (-27.992, -17.1524) -> (-28.0079, -18.8092)
  line L795 (-25.1908, -20.0079) -> (-24.008, -18.8476)
  line L796 (-34.8476, -19.992) -> (-33.1908, -20.0079)
  line L797 (-32.008, -18.8476) -> (-31.9921, -17.1908)
  line L798 (-31.9921, -17.1908) -> (-33.1524, -16.008)
  line L799 (-36.0079, -18.8092) -> (-34.8476, -19.992)
  line L800 (-33.1524, -16.008) -> (-34.8092, -15.9921)
  line L801 (-34.8092, -15.9921) -> (-35.992, -17.1524)
  line L802 (-35.992, -17.1524) -> (-36.0079, -18.8092)
  line L803 (-33.1908, -20.0079) -> (-32.008, -18.8476)
  line L804 (-42.8476, -19.992) -> (-41.1908, -20.0079)
  line L805 (-40.008, -18.8476) -> (-39.9921, -17.1908)
  line L806 (-39.9921, -17.1908) -> (-41.1524, -16.008)
  line L807 (-44.0079, -18.8092) -> (-42.8476, -19.992)
  line L808 (-41.1524, -16.008) -> (-42.8092, -15.9921)
  line L809 (-42.8092, -15.9921) -> (-43.992, -17.1524)
  line L810 (-43.992, -17.1524) -> (-44.0079, -18.8092)
  line L811 (-41.1908, -20.0079) -> (-40.008, -18.8476)
  line L812 (-50.8476, -19.992) -> (-49.1908, -20.0079)
  line L813 (-48.008, -18.8476) -> (-47.9921, -17.1908)
  line L814 (-47.9921, -17.1908) -> (-49.1524, -16.008)
  line L815 (-52.0079, -18.8092) -> (-50.8476, -19.992)
  line L816 (-49.1524, -16.008) -> (-50.8092, -15.9921)
  line L817 (-50.8092, -15.9921) -> (-51.992, -17.1524)
  line L818 (-51.992, -17.1524) -> (-52.0079, -18.8092)
  line L819 (-49.1908, -20.0079) -> (-48.008, -18.8476)
  line L820 (-58.8476, -19.992) -> (-57.1908, -20.0079)
  line L821 (-56.008, -18.8476) -> (-55.9921, -17.1908)
  line L822 (-55.9921, -17.1908) -> (-57.1524, -16.008)
  line L823 (-60.0079, -18.8092) -> (-58.8476, -19.992)
  line L824 (-57.1524, -16.008) -> (-58.8092, -15.9921)
  line L825 (-58.8092, -15.9921) -> (-59.992, -17.1524)
  line L826 (-59.992, -17.1524) -> (-60.0079, -18.8092)
  line L827 (-57.1908, -20.0079) -> (-56.008, -18.8476)
  line L828 (-66.8476, -19.992) -> (-65.1908, -20.0079)
  line L829 (-64.008, -18.8476) -> (-63.9921, -17.1908)
  line L830 (-63.9921, -17.1908) -> (-65.1524, -16.008)
  line L831 (-68.0079, -18.8092) -> (-66.8476, -19.992)
  line L832 (-65.1524, -16.008) -> (-66.8092, -15.9921)
  line L833 (-66.8092, -15.9921) -> (-67.992, -17.1524)
  line L834 (-67.992, -17.1524) -> (-68.0079, -18.8092)
  line L835 (-65.1908, -20.0079) -> (-64.008, -18.8476)
  line L836 (-74.8476, -19.992) -> (-73.1908, -20.0079)
  line L837 (-72.008, -18.8476) -> (-71.9921, -17.1908)
  line L838 (-71.9921, -17.1908) -> (-73.1524, -16.008)
  line L839 (-76.0079, -18.8092) -> (-74.8476, -19.992)
  line L840 (-73.1524, -16.008) -> (-74.8092, -15.9921)
  line L841 (-74.8092, -15.9921) -> (-75.992, -17.1524)
  line L842 (-75.992, -17.1524) -> (-76.0079, -18.8092)
  line L843 (-73.1908, -20.0079) -> (-72.008, -18.8476)
  line L844 (-82.8476, -19.992) -> (-81.1908, -20.0079)
  line L845 (-80.008, -18.8476) -> (-79.9921, -17.1908)
  line L846 (-79.9921, -17.1908) -> (-81.1524, -16.008)
  line L847 (-84.0079, -18.8092) -> (-82.8476, -19.992)
  line L848 (-81.1524, -16.008) -> (-82.8092, -15.9921)
  line L849 (-82.8092, -15.9921) -> (-83.992, -17.1524)
  line L850 (-83.992, -17.1524) -> (-84.0079, -18.8092)
  line L851 (-81.1908, -20.0079) -> (-80.008, -18.8476)
  line L852 (-90.8476, -19.992) -> (-89.1908, -20.0079)
  line L853 (-88.008, -18.8476) -> (-87.9921, -17.1908)
  line L854 (-87.9921, -17.1908) -> (-89.1524, -16.008)
  line L855 (-92.0079, -18.8092) -> (-90.8476, -19.992)
  line L856 (-89.1524, -16.008) -> (-90.8092, -15.9921)
  line L857 (-90.8092, -15.9921) -> (-91.992, -17.1524)
  line L858 (-91.992, -17.1524) -> (-92.0079, -18.8092)
  line L859 (-89.1908, -20.0079) -> (-88.008, -18.8476)
  line L860 (-98.8476, -19.992) -> (-97.1908, -20.0079)
  line L861 (-96.008, -18.8476) -> (-95.9921, -17.1908)
  line L862 (-95.9921, -17.1908) -> (-97.1524, -16.008)
  line L863 (-100.0079, -18.8092) -> (-98.8476, -19.992)
  line L864 (-97.1524, -16.008) -> (-98.8092, -15.9921)
  line L865 (-98.8092, -15.9921) -> (-99.992, -17.1524)
  line L866 (-99.992, -17.1524) -> (-100.0079, -18.8092)
  line L867 (-97.1908, -20.0079) -> (-96.008, -18.8476)
  line L868 (-106.8476, -19.992) -> (-105.1908, -20.0079)
  line L869 (-104.008, -18.8476) -> (-103.9921, -17.1908)
  line L870 (-103.9921, -17.1908) -> (-105.1524, -16.008)
  line L871 (-108.0079, -18.8092) -> (-106.8476, -19.992)
  line L872 (-105.1524, -16.008) -> (-106.8092, -15.9921)
  line L873 (-106.8092, -15.9921) -> (-107.992, -17.1524)
  line L874 (-107.992, -17.1524) -> (-108.0079, -18.8092)
  line L875 (-105.1908, -20.0079) -> (-104.008, -18.8476)
  line L876 (-114.8476, -19.992) -> (-113.1908, -20.0079)
  line L877 (-112.008, -18.8476) -> (-111.9921, -17.1908)
  line L878 (-111.9921, -17.1908) -> (-113.1524, -16.008)
  line L879 (-116.0079, -18.8092) -> (-114.8476, -19.992)
  line L880 (-113.1524, -16.008) -> (-114.8092, -15.9921)
  line L881 (-114.8092, -15.9921) -> (-115.992, -17.1524)
  line L882 (-115.992, -17.1524) -> (-116.0079, -18.8092)
  line L883 (-113.1908, -20.0079) -> (-112.008, -18.8476)
  line L884 (-122.8476, -19.992) -> (-121.1908, -20.0079)
  line L885 (-120.008, -18.8476) -> (-119.9921, -17.1908)
  line L886 (-119.9921, -17.1908) -> (-121.1524, -16.008)
  line L887 (-124.0079, -18.8092) -> (-122.8476, -19.992)
  line L888 (-121.1524, -16.008) -> (-122.8092, -15.9921)
  line L889 (-122.8092, -15.9921) -> (-123.992, -17.1524)
  line L890 (-123.992, -17.1524) -> (-124.0079, -18.8092)
  line L891 (-121.1908, -20.0079) -> (-120.008, -18.8476)
  line L892 (-130.8476, -19.992) -> (-129.1908, -20.0079)
  line L893 (-128.008, -18.8476) -> (-127.9921, -17.1908)
  line L894 (-127.9921, -17.1908) -> (-129.1524, -16.008)
  line L895 (-132.0079, -18.8092) -> (-130.8476, -19.992)
  line L896 (-129.1524, -16.008) -> (-130.8092, -15.9921)
  line L897 (-130.8092, -15.9921) -> (-131.992, -17.1524)
  line L898 (-131.992, -17.1524) -> (-132.0079, -18.8092)
  line L899 (-129.1908, -20.0079) -> (-128.008, -18.8476)
  line L900 (-138.8476, -19.992) -> (-137.1908, -20.0079)
  line L901 (-136.008, -18.8476) -> (-135.9921, -17.1908)
  line L902 (-135.9921, -17.1908) -> (-137.1524, -16.008)